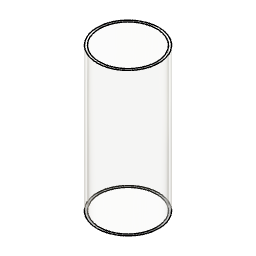
radhika (Autodesk Fusion 360 archive; units mm, degrees)
design "Prachi Proto Main Body"
Autodesk Fusion 360 part; units mm, degrees
sketch "Sketch1" plane through (0, 0, 0) normal (0, 1, 0) x (1, 0, 0)
  circle A0 centre (0, 0) radius 20
  circle A1 centre (0, 0) radius 21.5
  dimension "d1" = 40
  dimension "d2" = 1.5
  constraint coincident A0.centre A1.centre
  measures "d1" diameter of A0
extrude "Extrude1" add sketch "Sketch1" along normal blind 100

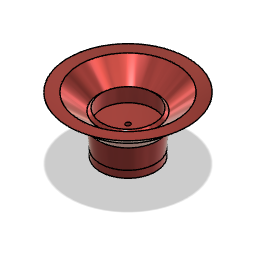
design "Prachi Proto Base Plate"
Autodesk Fusion 360 part; units mm, degrees
sketch "Sketch1" plane through (0, 0, 0) normal (0, 1, 0) x (1, 0, 0)
  circle A0 centre (0, 0) radius 18.5
  circle A1 centre (0, 0) radius 20
  dimension "d1" = 37
  dimension "d2" = 1.5
  constraint coincident A0.centre A1.centre
  measures "d1" diameter of A0
extrude "Extrude1" add sketch "Sketch1" along normal blind 15 draft 5 and the other way blind 5
sketch "Sketch2" plane through (0, 15, 0) normal (0, 1, 0) x (-1, 0, 0)
  circle A0 centre (0, 0) radius 17.1877
  circle A1 centre (0, 0) radius 21.3123
  circle A2 centre (0, 0) radius 17.1877
  circle A3 centre (0, 0) radius 21.3123
  constraint coincident A0.centre A1.centre
extrude "Extrude2" add sketch "Sketch2" along normal blind 10 draft 45
sketch "Sketch3" plane through (0, 25, 0) normal (0, 1, 0) x (-1, 0, 0)
  circle A0 centre (0, 0) radius 7.1877
  circle A1 centre (0, 0) radius 31.3123
  circle A2 centre (0, 0) radius 12.1877
  circle A3 centre (0, 0) radius 26.3123
  constraint concentric A0 A2
  constraint concentric A2 A3
extrude "Extrude3" add sketch "Sketch3" along normal blind 10 draft 50 contours A1 | A3
sketch "Sketch4" plane through (0, 25, 0) normal (0, 1, 0) x (-1, 0, 0)
  circle A0 centre (0, 0) radius 12.1877
  circle A1 centre (0, 0) radius 7.1877
  circle A2 centre (0, 0) radius 7.1877
  constraint coincident A0.centre A1.centre
extrude "Extrude4" cut sketch "Sketch4" along normal blind 60 contours A1 A2
sketch "Sketch5" plane through (0, 35, 0) normal (0, 1, 0) x (-1, 0, 0)
  circle A0 centre (0, 0) radius 7.1877
  circle A1 centre (0, 0) radius 43.2299
  circle A2 centre (0, 0) radius 35
  constraint coincident A0.centre A1.centre
extrude "Extrude5" cut sketch "Sketch5" against normal blind 20 draft -50 contours A2
ref_plane "WorkPlane1" through (0, 15, 0) normal (0, 1, 0) x (0, 0, 1)
sketch "Sketch6" plane through (0, 15, 0) normal (0, 1, 0) x (1, 0, 0)
  circle A0 centre (0, 0) radius 19
  dimension "d16" = 38
  constraint coincident A0.centre origin
  measures "d16" diameter of A0
extrude "Extrude6" cut sketch "Sketch6" along normal blind -70 and the other way blind -65
sketch "Sketch7" plane through (0, 15, 0) normal (0, 1, 0) x (1, 0, 0)
  circle A0 centre (0, 0) radius 19
  constraint coincident A0.centre origin
extrude "Extrude7" add sketch "Sketch7" against normal blind 15
sketch "Sketch8" plane through (0, 0, 0) normal (0, -1, 0) x (1, 0, 0)
  circle A0 centre (0, 0) radius 19
  circle A1 centre (0, 0) radius 19
  constraint concentric A0 A1
extrude "Extrude8" add sketch "Sketch8" along normal blind 10 draft -60
sketch "Sketch9" plane through (0, -10, 0) normal (0, -1, 0) x (1, 0, 0)
  circle A0 centre (0, 0) radius 1.6795
  circle A1 centre (0, 0) radius 1.6795
  dimension "d27" = 3.359
  constraint coincident A0.centre A1.centre
  measures "d27" diameter of A1
extrude "Extrude9" cut sketch "Sketch9" against normal blind 60
